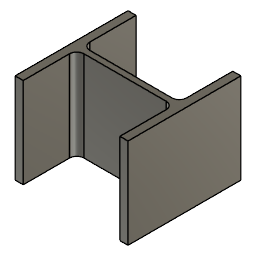
H-125×125×6.5×9 (Autodesk Fusion 360 design; units mm, degrees)
Autodesk Fusion 360 part; units mm, degrees
sketch "スケッチ1" plane through (0, 0, 0) normal (0, 0, 1) x (1, 0, 0)
  line L0 (0, 62.5) -> (0, -62.5)
  line L1 (125, -62.5) -> (125, 62.5)
  line L2 (17, -3.25) -> (108, -3.25)
  line L3 (9, -62.5) -> (9, -11.25)
  line L4 (0, -62.5) -> (9, -62.5)
  line L5 (116, -11.25) -> (116, -62.5)
  line L6 (116, -62.5) -> (125, -62.5)
  line L7 (108, 3.25) -> (17, 3.25)
  line L8 (9, 11.25) -> (9, 62.5)
  line L9 (9, 62.5) -> (0, 62.5)
  line L10 (116, 62.5) -> (116, 11.25)
  line L11 (125, 62.5) -> (116, 62.5)
  arc A0 (17, -3.25) -> (9, -11.25) centre (17, -11.25) ccw
  arc A1 (9, 11.25) -> (17, 3.25) centre (17, 11.25) ccw
  arc A2 (108, 3.25) -> (116, 11.25) centre (108, 11.25) ccw
  arc A3 (116, -11.25) -> (108, -3.25) centre (108, -11.25) ccw
extrude "押し出し1" add sketch "スケッチ1" along normal blind 100
